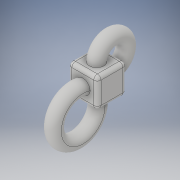
# Autodesk Inventor part: Lauren's funky piece
Saved by Autodesk Inventor 2017 (Build 210142000, 142)
## iProperties
Created: 2017-05-20
Part Number: Lauren's funky piece
Material: Generic
Document SubType Name: Modeling
Designer: User
Density: 1 g/cm^3
Appearance: Default
Author: User
Autodesk Inventor part; units mm, degrees
ref_plane "YZ Plane" through (0, 0, 0) normal (1, 0, 0) x (0, 1, 0)
ref_plane "XZ Plane" through (0, 0, 0) normal (0, 1, 0) x (-1, 0, 0)
sketch "Sketch1" plane through (0, 0, 0) normal (0, 0, 1) x (1, 0, 0)
  line L0 (0, 0) -> (25.4, 0)
  line L1 (25.4, 0) -> (25.4, 25.4)
  line L2 (25.4, 25.4) -> (0, 25.4)
  line L3 (0, 25.4) -> (0, 0)
  dimension "d0" = 25.4
  dimension "d1" = 25.4
  constraints: 8 end point, 2 parallel, 1 horizontal, 1 perpendicular
  measures "d0" distance of L2.end L1.end
  measures "d1" distance of L1.end L0.end
extrude "Extrusion1" add sketch "Sketch1" along normal blind 25.4
sketch "Sketch2" plane through (0, 25.4, 0) normal (0, 1, 0) x (1, 0, 0)
  line L0 (0, 0) -> (0, -25.4) projected
  line L1 (25.4, -25.4) -> (0, -25.4) projected
  circle A0 centre (12.7, -12.7) radius 6.35
  dimension "d4" = 12.7
  dimension "d5" = 12.7
  dimension "d6" = 12.7
  constraints: 1 centre point, 1 coincident
  measures "d4" distance from line of L0 point (12.7, -12.7)
  measures "d5" distance from line of L1 point (12.7, -12.7)
  measures "d6" diameter of A0
sketch "Sketch3" plane through (0, 0, 25.4) normal (0, 0, 1) x (1, 0, 0)
  line L0 (25.4, 25.4) -> (0, 25.4) projected
  line L1 (0, 25.4) -> (0, 0) projected
  circle A0 centre (12.7, 12.7) radius 6.35
  dimension "d7" = 12.7
  dimension "d8" = 12.7
  dimension "d9" = 12.7
  constraints: 1 centre point, 1 coincident
  measures "d7" distance from line of L0 point (12.7, 12.7)
  measures "d8" distance from line of L1 point (12.7, 12.7)
  measures "d9" diameter of A0
sketch "Sketch4" plane through (0, 0, 0) normal (0, -1, 0) x (1, 0, 0)
  line L0 (25.4, 0) -> (25.4, 25.4) projected
  line L1 (0, 25.4) -> (25.4, 25.4) projected
  circle A0 centre (12.7, 12.7) radius 6.35
  point P0 (0, 0)
  dimension "d10" = 12.7
  dimension "d11" = 12.7
  dimension "d12" = 12.7
  constraints: 1 centre point, 1 coincident
  measures "d10" distance from line of L0 point (12.7, 12.7)
  measures "d11" distance from line of L1 point (12.7, 12.7)
  measures "d12" diameter of A0
sketch "Sketch5" plane through (0, 0, 0) normal (0, 0, -1) x (-1, 0, 0)
  line L0 (-25.4, 0) -> (-25.4, 25.4) projected
  line L1 (0, 0) -> (-25.4, 0) projected
  circle A0 centre (-12.7, 12.7) radius 6.35
  dimension "d13" = 12.7
  dimension "d14" = 12.7
  dimension "d15" = 12.7
  constraints: 1 centre point, 1 coincident
  measures "d13" distance from line of point (-12.7, 12.7) L0
  measures "d14" distance from line of L1 point (-12.7, 12.7)
  measures "d15" diameter of A0
ref_plane "Work Plane1" through (12.7, 12.7, 25.4) normal (1, 0, 0) x (0, 0, -1)
sketch "Sketch6" plane through (12.7, 12.7, 25.4) normal (1, 0, 0) x (0, 0, -1)
  line L0 (25.4, -12.7) -> (25.4, 12.7) projected
  arc A0 (25.4, 0) -> (12.7731, 12.6779) centre (7.1702, -5.5295) ccw
  arc A1 (25.4, 0) -> (12.7731, 12.6779) centre (25.4731, 12.6998) ccw
  arc A2 (0, 0) -> (12.3568, -13.1392) centre (-6.0452, -18.0654) ccw
  dimension "d17" = 19.05
  dimension "d18" = 12.7
  dimension "d19" = 19.05
  constraints: 6 point on circle, 3 centre point, 1 midpoint
  measures "d17" radius of A0
  measures "d18" radius of A1
  measures "d19" radius of A2
sweep "Sweep1" add profiles "Sketch3" path "Sketch6" path curves A2
sketch "Sketch7" plane through (12.7, 12.7, 25.4) normal (1, 0, 0) x (0, 0, -1)
  arc A0 (25.3272, -0.0369) -> (12.0094, 12.137) centre (24.6991, 12.6475) ccw
  point P0 (25.4, -12.7)
  dimension "d23" = 12.7
  constraints: 2 point on circle, 1 centre point
  measures "d23" radius of A0
sweep "Sweep2" add profiles "Sketch5" path "Sketch7"
fillet "Fillet1" radius 3.175 1 edges at (25.4, 25.4, 12.7)
fillet "Fillet2" radius 3.175 3 edges at (24.4701, 24.4701, 0) (11.1125, 25.4, 0) (25.4, 11.1125, 0)
fillet "Fillet3" radius 3.175 3 edges at (24.4701, 24.4701, 25.4) (11.1125, 25.4, 25.4) (25.4, 11.1125, 25.4)
fillet "Fillet4" radius 3.175 5 edges at (24.4701, 0, 24.4701) (11.1125, 0, 25.4) (24.4701, 0, 0.9299) (11.1125, 0, 0) (25.4, 0, 12.7)
fillet "Fillet5" radius 3.175 8 edges at (0, 0.9299, 24.4701) (0, 12.7, 25.4) (0, 24.4701, 24.4701) (0, 25.4, 12.7) (0, 24.4701, 0.9299) (0, 12.7, 0) (0, 0.9299, 0.9299) (0, 0, 12.7)
body "Solid1"
